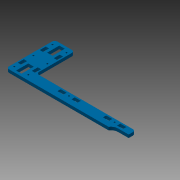
# Autodesk Inventor part: zCar_a
Saved by Autodesk Inventor 2013 (Build 170138000, 138)
## iProperties
Created: 2015-01-14
Part Number: zCar_a
Material: Generic
Document SubType Name: Modeling
Designer: dzban
Density: 1 g/cm^3
Author: dzban
Autodesk Inventor part; units mm, degrees
ref_plane "YZ Plane" through (0, 0, 0) normal (1, 0, 0) x (0, 1, 0)
ref_plane "XZ Plane" through (0, 0, 0) normal (0, 1, 0) x (-1, 0, 0)
ref_plane "XY Plane" through (0, 0, 0) normal (0, 0, 1) x (1, 0, 0)
sketch "Sketch1" plane through (0, 0, 0) normal (0, 0, 1) x (1, 0, 0)
  line L0 (196.0836, -19.606) -> (216.6625, -19.606)
  arc A0 (216.6625, -19.606) -> (216.9836, -17.2233) centre (207.9836, -17.2233) ccw
  line L1 (216.9836, -17.2233) -> (216.9836, -11.2233)
  arc A1 (216.9836, -11.2233) -> (211.9836, -6.2233) centre (211.9836, -11.2233) ccw
  line L2 (211.9836, -6.2233) -> (26.9836, -6.2233)
  arc A2 (21.9836, -1.2233) -> (26.9836, -6.2233) centre (26.9836, -1.2233) ccw
  line L3 (21.9836, -1.2233) -> (21.9836, 63.7767)
  arc A3 (21.9836, 63.7767) -> (16.9836, 68.7767) centre (16.9836, 63.7767) ccw
  line L4 (16.9836, 68.7767) -> (-12.0164, 68.7767)
  arc A4 (-12.0164, 68.7767) -> (-17.0164, 63.7767) centre (-12.0164, 63.7767) ccw
  line L5 (-17.0164, 63.7767) -> (-17.0164, -21.2233)
  arc A5 (-17.0164, -21.2233) -> (-12.0164, -26.2233) centre (-12.0164, -21.2233) ccw
  line L6 (-12.0164, -26.2233) -> (184.2764, -26.2233)
  arc A6 (196.0836, -19.606) -> (184.2764, -26.2233) centre (196.0836, -33.4483) ccw
  circle A7 centre (-11.3164, 21.2767) radius 1.5
  circle A8 centre (16.2836, 21.2767) radius 1.5
  circle A9 centre (16.2836, -16.2233) radius 1.5
  circle A10 centre (-11.3164, -16.2233) radius 1.5
  circle A11 centre (92.5836, -12.4233) radius 1.5
  circle A12 centre (182.1836, -12.4233) radius 1.5
  circle A13 centre (-11.3164, 58.7767) radius 1.5
  circle A14 centre (16.2836, 58.7767) radius 1.5
  line L7 (13.0836, 36.9767) -> (13.0836, 48.7767)
  line L8 (13.0836, 48.7767) -> (19.4836, 48.7767)
  line L9 (19.4836, 48.7767) -> (19.4836, 36.9767)
  line L10 (19.4836, 36.9767) -> (13.0836, 36.9767)
  line L11 (-8.1164, 48.7767) -> (-8.1164, 36.9767)
  line L12 (-8.1164, 36.9767) -> (-14.5164, 36.9767)
  line L13 (-14.5164, 36.9767) -> (-14.5164, 48.7767)
  line L14 (-14.5164, 48.7767) -> (-8.1164, 48.7767)
  line L15 (13.0836, -6.2233) -> (13.0836, 5.5767)
  line L16 (13.0836, 5.5767) -> (19.4836, 5.5767)
  line L17 (19.4836, 5.5767) -> (19.4836, -6.2233)
  line L18 (19.4836, -6.2233) -> (13.0836, -6.2233)
  line L19 (201.9836, -9.2233) -> (201.9836, -15.6233)
  line L20 (201.9836, -15.6233) -> (190.1836, -15.6233)
  line L21 (190.1836, -15.6233) -> (190.1836, -9.2233)
  line L22 (190.1836, -9.2233) -> (201.9836, -9.2233)
  line L23 (174.1836, -9.2233) -> (174.1836, -15.6233)
  line L24 (174.1836, -15.6233) -> (162.3836, -15.6233)
  line L25 (162.3836, -15.6233) -> (162.3836, -9.2233)
  line L26 (162.3836, -9.2233) -> (174.1836, -9.2233)
  line L27 (112.3836, -9.2233) -> (112.3836, -15.6233)
  line L28 (112.3836, -15.6233) -> (100.5836, -15.6233)
  line L29 (100.5836, -15.6233) -> (100.5836, -9.2233)
  line L30 (100.5836, -9.2233) -> (112.3836, -9.2233)
  line L31 (84.5836, -9.2233) -> (84.5836, -15.6233)
  line L32 (84.5836, -15.6233) -> (72.7836, -15.6233)
  line L33 (72.7836, -15.6233) -> (72.7836, -9.2233)
  line L34 (72.7836, -9.2233) -> (84.5836, -9.2233)
  line L35 (-8.1164, 5.5767) -> (-8.1164, -6.2233)
  line L36 (-8.1164, -6.2233) -> (-14.5164, -6.2233)
  line L37 (-14.5164, -6.2233) -> (-14.5164, 5.5767)
  line L38 (-14.5164, 5.5767) -> (-8.1164, 5.5767)
  line L39 (7.8336, 63.7767) -> (7.8336, 39.7767)
  line L40 (7.8336, 39.7767) -> (-2.8664, 39.7767)
  line L41 (-2.8664, 39.7767) -> (-2.8664, 63.7767)
  line L42 (-2.8664, 63.7767) -> (7.8336, 63.7767)
  line L43 (7.8336, 2.7767) -> (7.8336, -21.2233)
  line L44 (7.8336, -21.2233) -> (-2.8664, -21.2233)
  line L45 (-2.8664, -21.2233) -> (-2.8664, 2.7767)
  line L46 (-2.8664, 2.7767) -> (7.8336, 2.7767)
  point P0 (0, 0)
  point P1 (0, 0)
  constraints: 94 end point, 15 centre point, 14 point on circle
extrude "Extrusion1" add sketch "Sketch1" along normal blind 6
body "Solid1"
